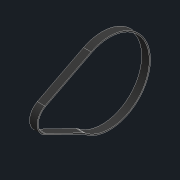
# Autodesk Inventor part: belt_2
Saved by Autodesk Inventor 2022 (Build 260153000, 153)
## iProperties
Created: 2021-07-18
Part Number: belt_2
Material: ゴム
Document SubType Name: Modeling
Designer: yuta0
Density: 0.93 g/cm^3
Appearance: ゴム - 黒
Mass: 8.55769 g
Surface Area: 248.449 cm^2
Volume: 9.20182 cm^3
購入先: ミスミ
在庫数: 0.0
Author: yuta0
Autodesk Inventor part; units mm, degrees
ref_plane "YZ Plane" through (0, 0, 0) normal (1, 0, 0) x (0, 1, 0)
ref_plane "XZ Plane" through (0, 0, 0) normal (0, 1, 0) x (-1, 0, 0)
ref_plane "XY Plane" through (0, 0, 0) normal (0, 0, 1) x (1, 0, 0)
sketch "スケッチ1" plane through (0, 0, 0) normal (1, 0, 0) x (0, 1, 0)
  arc A0 (15.5817, 7.9817) -> (-15.7529, 7.6382) centre (0, 0) ccw
  arc A1 (-41.5342, -44.6538) -> (46.7451, -52.855) centre (0, -76.8) ccw
  arc A2 (-40.9669, -43.9208) -> (-39.9838, -42.3353) centre (-48.1, -38.4) ccw
  line L0 (-39.9838, -42.3353) -> (-15.7529, 7.6382)
  line L1 (46.7451, -52.855) -> (15.5817, 7.9817)
  line L2 (-40.9669, -43.9208) -> (-41.5342, -44.6538)
  arc A3 (16.4895, 8.4467) -> (-16.6707, 8.0832) centre (0, 0) ccw
  line L3 (-16.6707, 8.0832) -> (-40.9016, -41.8903)
  arc A4 (-41.7735, -43.2965) -> (-40.9016, -41.8903) centre (-48.1, -38.4) ccw
  line L4 (-41.7735, -43.2965) -> (-42.3409, -44.0295)
  arc A5 (-42.3409, -44.0295) -> (47.6529, -52.3899) centre (0, -76.8) ccw
  line L5 (47.6529, -52.3899) -> (16.4895, 8.4467)
  arc A6 (15.1545, 7.7628) -> (-15.321, 7.4288) centre (0, 0) ccw
  line L6 (-15.321, 7.4288) -> (-39.5518, -42.5448)
  arc A7 (-40.5873, -44.2146) -> (-39.5518, -42.5448) centre (-48.1, -38.4) ccw
  line L7 (-40.5873, -44.2146) -> (-41.1546, -44.9476)
  arc A8 (-41.1546, -44.9476) -> (46.3179, -53.0738) centre (0, -76.8) ccw
  line L8 (46.3179, -53.0738) -> (15.1545, 7.7628)
  dimension "d0" = 35.0141
  dimension "d1" = 105.0423
  dimension "d2" = 76.8
  dimension "d25" = 8
  dimension "d26" = 38.4
  dimension "d30" = 48.1
  dimension "d31" = 1.5
  dimension "d32" = 0.48
  constraints: 18 end point, 18 point on circle, 9 centre point, 6 tangent, 1 coincident, 1 vertical alignment, 10 other
  measures "d0" diameter of A0
  measures "d1" diameter of A1
  measures "d2" distance of A0.centre A1.centre
  measures "d25" radius of A4
  measures "d26" vertical distance of point (0, 0) A2.centre
  measures "d30" horizontal distance of point (0, 0) A2.centre
  measures "d31" distance between parallel lines of L5 L8
  measures "d32" distance between parallel lines of L8 L1
extrude "押し出し1" add sketch "スケッチ1" along normal mid plane 10 contours L1 A1 L2 A2 L0 A0 | L5 A5 L4 A4 L3 A3
equation "\"d26\" = 0.5 * d2"
